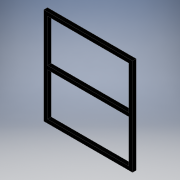
# Autodesk Inventor part: Pool Door
Saved by Autodesk Inventor 2016 (Build 200138000, 138)
## iProperties
Created: 2015-07-05
Part Number: Pool Door
Material: Aluminum 6061
Document SubType Name: Modeling
Designer: steele
Density: 2.7 g/cm^3
Appearance: Black
Author: steele
Autodesk Inventor part; units mm, degrees
ref_plane "YZ Plane" through (0, 0, 0) normal (1, 0, 0) x (0, 1, 0)
ref_plane "XZ Plane" through (0, 0, 0) normal (0, 1, 0) x (-1, 0, 0)
ref_plane "XY Plane" through (0, 0, 0) normal (0, 0, 1) x (1, 0, 0)
sketch "Sketch1" plane through (0, 0, 0) normal (0, 0, 1) x (1, 0, 0)
  line L0 (-609.6, -663.575) -> (609.6, -663.575)
  line L1 (609.6, -663.575) -> (609.6, 663.575)
  line L2 (609.6, 663.575) -> (-609.6, 663.575)
  line L3 (-609.6, 663.575) -> (-609.6, -663.575)
  line L4 (-609.6, -663.575) -> (609.6, 663.575) construction
  line L5 (609.6, -663.575) -> (-609.6, 663.575) construction
  line L6 (-558.8, -612.775) -> (558.8, -612.775)
  line L7 (558.8, -612.775) -> (558.8, 612.775)
  line L8 (558.8, 612.775) -> (-558.8, 612.775)
  line L9 (-558.8, 612.775) -> (-558.8, -612.775)
  line L10 (-558.8, -612.775) -> (558.8, 612.775) construction
  line L11 (558.8, -612.775) -> (-558.8, 612.775) construction
  line L12 (-558.8, -25.4) -> (558.8, -25.4)
  line L13 (558.8, -25.4) -> (558.8, 25.4)
  line L14 (558.8, 25.4) -> (-558.8, 25.4)
  line L15 (-558.8, 25.4) -> (-558.8, -25.4)
  line L16 (-558.8, -25.4) -> (558.8, 25.4) construction
  line L17 (558.8, -25.4) -> (-558.8, 25.4) construction
  point P0 (0, 0)
  dimension "d0" = 1219.2
  dimension "height" = 1327.15
  dimension "d2" = 1117.6
  dimension "d3" = 1225.55
  dimension "d4" = 50.8
  constraints: 36 end point, 7 parallel, 6 midpoint, 3 perpendicular, 2 horizontal
  measures "d0" distance of L1.end L2.end
  measures "height" distance of L0.end L1.end
  measures "d2" distance of L6.start L6.end
  measures "d3" distance of L8.end L6.start
  measures "d4" distance between parallel lines of L12 L14
extrude "Extrusion1" add sketch "Sketch1" along normal mid plane 50.8 contours L3 L2 L1 L0 | L9 L14 L7 L12
body "Solid1"
